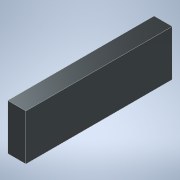
# Autodesk Inventor part: akksi
Saved by Autodesk Inventor 2022 (Build 260153000, 153)
## iProperties
Created: 2021-10-06
Part Number: akksi
Material: Iron, Cast
Document SubType Name: Modeling
Designer: Varga Tamás
Mass: 716.051 g
Surface Area: 179.02 cm^2
Volume: 100.147 cm^3
Density: 7.15 g/cm^3
Appearance: Iron Gray
Author: Varga Tamás
Autodesk Inventor part; units mm, degrees
ref_plane "YZ Plane" through (0, 0, 0) normal (1, 0, 0) x (0, 1, 0)
ref_plane "XZ Plane" through (0, 0, 0) normal (0, 1, 0) x (-1, 0, 0)
ref_plane "XY Plane" through (0, 0, 0) normal (0, 0, 1) x (1, 0, 0)
sketch "Sketch1" plane through (0, 0, 0) normal (0, 1, 0) x (-1, 0, 0)
  line L0 (0, 0) -> (17, 0)
  line L1 (17, 0) -> (17, -137)
  line L2 (17, -137) -> (0, -137)
  line L3 (0, -137) -> (0, 0)
  dimension "d0" = 17
  dimension "d1" = 137
  constraints: 8 end point, 2 parallel, 1 horizontal, 1 perpendicular
  measures "d0" distance of L0.start L0.end
  measures "d1" distance of L0.end L1.end
extrude "Extrusion1" add sketch "Sketch1" along normal blind 43
body "Solid1"
